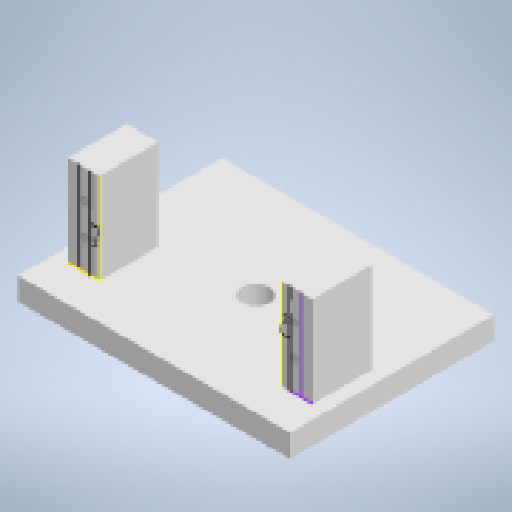
# Autodesk Inventor part: Part1
Saved by Autodesk Inventor 2025.2 (Build 292293000, 293)
## iProperties
Created: 2025-02-15
Part Number: Part1
Material: Generic
Document SubType Name: Modeling
Designer: maqmat
Density: 1 g/cm^3
Appearance: Default
Author: maqmat
Autodesk Inventor part; units mm, degrees
ref_plane "YZ Plane" through (0, 0, 0) normal (1, 0, 0) x (0, 1, 0)
ref_plane "XZ Plane" through (0, 0, 0) normal (0, 1, 0) x (-1, 0, 0)
ref_plane "XY Plane" through (0, 0, 0) normal (0, 0, 1) x (1, 0, 0)
sketch "Sketch1" plane through (0, 0, 0) normal (0, 1, 0) x (-1, 0, 0)
  line L0 (19.5703, 29.4197) -> (-40.4297, 29.4197)
  line L1 (-40.4297, 29.4197) -> (-40.4297, -15.5803)
  line L2 (-40.4297, -15.5803) -> (19.5703, -15.5803)
  line L3 (19.5703, -15.5803) -> (19.5703, 29.4197)
  point P0 (0, 0)
  dimension "d2" = 60
  dimension "d3" = 45
  constraints: 8 end point, 2 parallel, 1 horizontal, 1 perpendicular
  measures "d2" distance of L2.end L1.end
  measures "d3" distance of L1.end L0.end
extrude "Extrusion1" add sketch "Sketch1" along normal blind 5
sketch "Sketch2" plane through (0, 5, 0) normal (0, 1, 0) x (1, 0, 0)
  line L0 (-19.5703, 15.5803) -> (-19.5703, -29.4197) projected
  line L1 (40.4297, -29.4197) -> (40.4297, 15.5803) projected
  line L2 (-19.5703, -29.4197) -> (40.4297, -29.4197) projected
  line L3 (40.4297, 15.5803) -> (-19.5703, 15.5803) projected
  circle A0 centre (10.4297, -6.9197) radius 3
  point P0 (0, 0)
  point P1 (13.4635, -6.9197)
  constraints: 1 centre point, 1 coincident
extrude "Extrusion2" cut sketch "Sketch2" against normal up to next contours A0
sketch "Sketch3" plane through (0, 0, 0) normal (0, -1, 0) x (1, 0, 0)
  circle A0 centre (10.4297, 6.9197) radius 3 projected
  circle A1 centre (10.4297, 6.9197) radius 5
  point P0 (0, 0)
  dimension "d9" = 10
  constraints: 1 centre point, 1 coincident
  measures "d9" diameter of A1
extrude "Extrusion3" add sketch "Sketch3" along normal blind 10
sketch "Sketch6" plane through (0, 5, 0) normal (0, 1, 0) x (1, 0, 0)
  line L0 (-19.5703, -29.4197) -> (40.4297, -29.4197) projected
  line L1 (-19.5703, -29.4197) -> (-19.5703, -21.4197)
  line L2 (-19.5703, 15.5803) -> (-19.5703, -29.4197) projected
  line L3 (-19.5703, -21.4197) -> (40.4297, -21.4197)
  line L4 (40.4297, -29.4197) -> (40.4297, 15.5803) projected
  line L5 (10.4297, -29.4197) -> (10.4297, 15.5803)
  line L6 (40.4297, 15.5803) -> (-19.5703, 15.5803) projected
  line L7 (10.4297, -21.4197) -> (37.4297, -21.4197)
  line L8 (10.4297, -21.4197) -> (-16.5703, -21.4197)
  line L9 (-16.5703, -8.4197) -> (-9.5703, -8.4197)
  line L10 (37.4297, -21.4197) -> (37.4297, -8.4197)
  line L11 (37.4297, -8.4197) -> (30.4297, -8.4197)
  line L12 (30.4297, -8.4197) -> (30.4297, -21.4197)
  line L13 (-9.5703, -8.4197) -> (-9.5703, -21.4197)
  line L14 (-16.5703, -8.4197) -> (-16.5703, -21.4197)
  point P0 (0, 0)
  dimension "d22" = 8
  dimension "d23" = 27
  dimension "d24" = 27
  dimension "d25" = 13
  dimension "d26" = 7
  dimension "d27" = 13
  dimension "d28" = 7
  constraints: 22 end point, 9 point on line, 4 perpendicular, 2 midpoint
  measures "d22" distance of L0.start L1.end
  measures "d23" distance of L7.start L7.end
  measures "d24" distance of L7.start L8.end
  measures "d25" distance of L8.end L9.start
  measures "d26" distance of L9.start L9.end
  measures "d27" distance of L7.end L10.end
  measures "d28" distance of L10.end L11.end
extrude "Extrusion5" add sketch "Sketch6" along normal blind 20 contours L14 L9 L13 L3 | L12 L11 L10 L3
sketch "Sketch7" plane through (-16.5703, 5, 21.4197) normal (0, 0, 1) x (1, 0, 0)
  line L0 (7, 0) -> (7, 20) projected
  line L1 (7, 10) -> (5, 10)
  line L2 (5, 10) -> (5, 20)
  line L3 (5, 10) -> (5, 0)
  line L4 (7, 0) -> (0, 0) projected
  line L5 (0, 0) -> (5, 0)
  line L6 (2.5, 0) -> (2.5, 20)
  line L7 (47, 0) -> (47, 20) projected
  line L8 (47, 10) -> (49, 10)
  line L9 (49, 10) -> (49, 20)
  line L10 (49, 10) -> (49, 0)
  line L11 (49, 0) -> (53.9219, 0)
  line L12 (51.4609, 0) -> (51.4609, 20)
  point P0 (16.5703, -5)
  dimension "d31" = 2
  dimension "d32" = 2
  constraints: 20 end point, 4 midpoint, 4 vertical, 2 horizontal, 2 perpendicular, 1 collinear, 1 parallel
  measures "d31" distance of L1.start L1.end
  measures "d32" distance of L8.start L8.end
sketch "Sketch8" plane through (30.4297, 5, 21.4197) normal (0, 0, 1) x (1, 0, 0)
  line L0 (2.0988, 10) -> (3.0988, 10)
  line L1 (7, 0) -> (7, 20) projected
  line L2 (3.0988, 12.5) -> (3.0988, 13.5)
  line L3 (0, 0) -> (0, 20) projected
  circle A0 centre (3.0988, 13.5) radius 1
  line L4 (3.0988, 7.5) -> (3.0988, 6.5)
  circle A1 centre (3.0988, 6.5) radius 1
  line L5 (-42.0376, 10) -> (-43.0376, 10)
  line L6 (-43.0376, 12.5) -> (-43.0376, 13.5)
  line L7 (-43.0376, 7.5) -> (-43.0376, 6.5)
  circle A2 centre (-43.0376, 13.5) radius 1
  circle A3 centre (-43.0376, 6.5) radius 1
  point P0 (-30.4297, -5)
  constraints: 12 end point, 4 coincident, 4 vertical alignment, 2 horizontal, 1 parallel, 1 point on line, 1 vertical, 8 other
extrude "Extrusion6" cut sketch "Sketch8" against normal blind 14
thread "Thread1" size "M2x0.4" class "6H" standard "ANSI Metric M Profile" full length
thread "Thread2" size "M2x0.4" class "6H" standard "ANSI Metric M Profile" full length
thread "Thread3" size "M2x0.4" class "6H" standard "ANSI Metric M Profile" full length
thread "Thread4" size "M2x0.4" class "6H" standard "ANSI Metric M Profile" full length
sketch "Sketch9" plane through (-19.5703, 0, 29.4197) normal (0, 0, 1) x (1, 0, 0)
  line L0 (35, 0) -> (25, 0) projected
  line L1 (25, -10) -> (35, -10) projected
  line L2 (25, 0) -> (25, -10)
  line L3 (25, -10) -> (35, -10)
  line L4 (35, -10) -> (35, 0)
  line L5 (35, 0) -> (35, -10) projected
  point P0 (19.5703, 0)
  constraints: 6 end point, 1 collinear, 1 perpendicular, 1 point on line
extrude "Extrusion7" cut sketch "Sketch9" against normal blind 40
body "Solid1"
